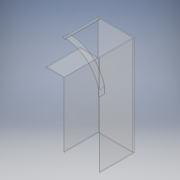
# Autodesk Inventor part: Sorter
Saved by Autodesk Inventor 2019 (Build 230136000, 136)
## iProperties
Created: 2018-11-20
Part Number: Sorter
Material: Polycarbonate, Clear
Document SubType Name: Modeling
Designer: User
Density: 1.2 g/cm^3
Appearance: Polycarbonate - Clear
Author: User
Autodesk Inventor part; units mm, degrees
ref_plane "YZ Plane" through (0, 0, 0) normal (1, 0, 0) x (0, 1, 0)
ref_plane "XZ Plane" through (0, 0, 0) normal (0, 1, 0) x (-1, 0, 0)
ref_plane "XY Plane" through (0, 0, 0) normal (0, 0, 1) x (1, 0, 0)
sketch "Sketch1" plane through (0, 0, 0) normal (0, 0, 1) x (1, 0, 0)
  line L0 (0, 0) -> (79.9084, 0)
  line L1 (79.9084, 0) -> (79.9084, 219.6084)
  line L2 (79.9084, 219.6084) -> (0, 219.6084)
  line L3 (0, 219.6084) -> (0, 0)
  dimension "d0" = 79.9084
  dimension "d1" = 219.6084
  constraints: 8 end point, 2 parallel, 1 horizontal, 1 perpendicular
  measures "d0" distance of L2.end L1.end
  measures "d1" distance between parallel lines of L2 L0
extrude "Extrusion1" add sketch "Sketch1" along normal blind 76.2
sketch "Sketch2" plane through (0, 0, 0) normal (0, -1, 0) x (1, 0, 0)
  line L0 (79.9084, 0) -> (79.9084, 76.2) projected
  line L1 (0, 0) -> (79.9084, 0) projected
  line L2 (0, 76.2) -> (79.9084, 76.2) projected
  line L3 (78.0542, 1.8542) -> (1.8542, 1.8542)
  line L4 (1.8542, 1.8542) -> (1.8542, 76.2)
  line L5 (1.8542, 76.2) -> (78.0542, 76.2)
  line L6 (78.0542, 76.2) -> (78.0542, 1.8542)
  dimension "d4" = 1.8542
  dimension "d5" = 1.8542
  dimension "d6" = 76.2
  constraints: 8 end point, 2 parallel, 1 horizontal, 1 perpendicular, 1 point on line
  measures "d4" distance from line of L0 L3.start
  measures "d5" distance from line of L1 L3.start
  measures "d6" distance of L4.end L5.end
extrude "Extrusion2" cut sketch "Sketch2" against normal blind 228.6
sketch "Sketch3" plane through (0, 0, 76.2) normal (0, 0, 1) x (1, 0, 0)
  line L0 (1.8542, 0) -> (1.8542, 219.6084) projected
  line L1 (0, 219.6084) -> (1.8542, 219.6084)
  line L2 (1.8542, 219.6084) -> (1.8542, 143.4084)
  line L3 (1.8542, 143.4084) -> (0, 143.4084)
  line L4 (0, 143.4084) -> (0, 219.6084)
  point P0 (0, 0)
  dimension "d9" = 76.2
  constraints: 8 end point, 2 parallel, 1 horizontal, 1 perpendicular, 1 point on line
  measures "d9" distance of L1.end L2.end
extrude "Extrusion3" cut sketch "Sketch3" against normal blind 74.3458
sketch "Sketch4" plane through (0, 0, 0) normal (-1, 0, 0) x (0, 0, 1)
  line L0 (76.2, 143.4084) -> (1.8542, 143.4084) projected
  line L1 (76.2, 0) -> (76.2, 143.4084) projected
  line L2 (1.8542, 143.4084) -> (76.2, 143.4084)
  line L3 (76.2, 143.4084) -> (76.2, 141.5542)
  line L4 (76.2, 141.5542) -> (1.8542, 141.5542)
  line L5 (1.8542, 141.5542) -> (1.8542, 143.4084)
  point P0 (0, 0)
  dimension "d12" = 1.8542
  constraints: 8 end point, 2 parallel, 1 horizontal, 1 perpendicular, 1 point on line
  measures "d12" distance of L2.end L3.end
extrude "Extrusion4" add sketch "Sketch4" along normal blind 38.1
sketch "Sketch6" plane through (0, 0, 76.2) normal (0, 0, 1) x (1, 0, 0)
  line L0 (79.9084, 0) -> (79.9084, 219.6084) projected
  arc A0 (79.9084, 143.4084) -> (0, 219.6084) centre (0.14, 139.7566) ccw
  line L1 (0, 219.6084) -> (0, 0) projected
  arc A1 (78.0076, 143.4084) -> (0, 217.7542) centre (0.9271, 140.6292) ccw
  line L2 (0, 217.7542) -> (0, 219.6084)
  line L3 (78.0076, 143.4084) -> (79.9084, 143.4084)
  line L4 (78.0542, 0) -> (78.0542, 219.6084) projected
  dimension "d15" = 1.8542
  constraints: 4 end point, 4 point on circle, 2 centre point, 2 point on line, 1 perpendicular, 1 vertical
  measures "d15" distance of L1.start L2.start
extrude "Extrusion5" add sketch "Sketch6" against normal blind 12.7
sketch "Sketch8" plane through (1.8542, 0, 1.8542) normal (0, 0, 1) x (1, 0, 0)
  line L0 (-1.8542, 217.6656) -> (3.2258, 217.6656)
  line L1 (-1.8542, 217.6656) -> (3.2258, 217.6656) construction
  line L2 (3.2258, 217.6656) -> (3.2258, 219.6084)
  line L3 (78.0542, 219.6084) -> (-1.8542, 219.6084) projected
  line L4 (3.2258, 219.6084) -> (-1.8542, 219.6084)
  line L5 (-1.8542, 219.6084) -> (-1.8542, 217.6656)
  point P0 (-1.8542, 0)
  dimension "d18" = 5.08
  dimension "d19" = 0
  constraints: 10 end point, 3 perpendicular, 2 horizontal, 1 collinear
  measures "d18" distance of L0.start L0.end
  measures "d19" distance between parallel lines of L0 L1
extrude "Extrusion6" add sketch "Sketch8" along normal blind 76.2
body "Solid1"
